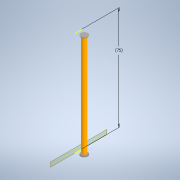
# Autodesk Inventor part: vint
Saved by Autodesk Inventor 2020 (Build 240168000, 168)
## iProperties
Created: 2022-07-20
Part Number: vint
Material: Типовые
Document SubType Name: Modeling
Designer: akapu
Density: 1 g/cm^3
Appearance: По умолчанию
Author: akapu
Autodesk Inventor part; units mm, degrees
ref_plane "YZ Plane" through (0, 0, 0) normal (1, 0, 0) x (0, 1, 0)
ref_plane "XZ Plane" through (0, 0, 0) normal (0, 1, 0) x (-1, 0, 0)
ref_plane "XY Plane" through (0, 0, 0) normal (0, 0, 1) x (1, 0, 0)
sketch "Эскиз1" plane through (0, 0, 0) normal (0, 1, 0) x (-1, 0, 0)
  circle A0 centre (0, 0) radius 1.6
  dimension "d0" = 3.2
  constraints: 1 centre point, 1 coincident
  measures "d0" diameter of A0
extrude "Выдавливание1" add sketch "Эскиз1" along normal blind 75
sketch "Эскиз2" plane through (0, 75, 0) normal (0, 1, 0) x (1, 0, 0)
  circle A0 centre (0, 0) radius 2.5
  dimension "d3" = 5
  constraints: 1 centre point, 1 coincident
  measures "d3" diameter of A0
extrude "Выдавливание2" add sketch "Эскиз2" against normal blind 1
fillet "Сопряжение1" radius 1 1 edges at (-2.5, 74, 0)
sketch "Эскиз3" plane through (0, 0, 0) normal (0, -1, 0) x (1, 0, 0)
  circle A0 centre (0, 0) radius 2.5
  constraints: 1 centre point, 1 coincident
extrude "Выдавливание3" add sketch "Эскиз3" against normal blind 1
fillet "Сопряжение2" radius 1 1 edges at (-2.5, 1, 0)
ref_plane "РабПлоскость1" through (-4.5, 3.005, 18.077) normal (-1, 0, 0) x (0, 0, -1)
sketch "Эскиз4" plane through (-4.5, 3.005, 18.077) normal (-1, 0, 0) x (0, 0, -1)
  line L0 (15.577, -71.995) -> (20.577, -71.995) projected
  line L1 (20.577, 3.005) -> (15.577, 3.005) projected
  point P0 (18.077, 3.005)
  dimension "d10" = 75
  measures "d10" distance between parallel lines of L0 L1
